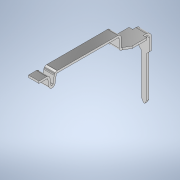
# Autodesk Inventor part: USB 3.0 A Recepticle Lower Pin
Saved by Autodesk Inventor 2020.1 (Build 241239000, 239)
## iProperties
Created: 2019-11-21
Part Number: USB 3.0 A Recepticle Lower Pin
Material: Nickel-Copper Alloy 400
Document SubType Name: Sheet Metal
Designer: S. Lee
Mass: 0.0317253 g
Surface Area: 0.43999 cm^2
Volume: 0.0035929 cm^3
Density: 8.83 g/cm^3
Appearance: Chrome - Polished
Flat Pattern Width: 0.17 cm
Flat Pattern Length: 1.89049 cm
Flat Pattern Area: 0.321383 cm^2
Sheet Metal Rule: Default_mm
Sheet Metal Width: 1.700 mm
Sheet Metal Length: 18.905 mm
Sheet Metal Area: 32.138 mm^2
Author: S. Lee
Autodesk Inventor part; units mm, degrees
ref_plane "YZ Plane" through (0, 0, 0) normal (1, 0, 0) x (0, 1, 0)
ref_plane "XZ Plane" through (0, 0, 0) normal (0, 1, 0) x (-1, 0, 0)
sketch "Sketch1" plane through (0, 0, 0) normal (1, 0, 0) x (0, 1, 0)
  line L0 (1.1156, 6.8012) -> (0.4531, 6.6963)
  line L1 (0.4531, 6.1037) -> (1.1156, 5.9988)
  line L2 (1.2, 5.9) -> (1.2, 0.1)
  line L3 (1.1, 0) -> (0.3, 0)
  line L4 (0, -0.3) -> (0, -2.6)
  line L5 (-0.3, -2.9) -> (-5.95, -2.9)
  line L6 (-5.95, -2.9) -> (-5.95, -3.1)
  line L7 (-5.95, -3.1) -> (-0.3, -3.1)
  line L8 (0.2, -2.6) -> (0.2, -0.3)
  line L9 (0.3, -0.2) -> (1.1, -0.2)
  line L10 (1.4, 0.1) -> (1.4, 5.9)
  line L11 (1.1469, 6.1963) -> (0.4844, 6.3012)
  line L12 (0.4844, 6.4988) -> (1.1469, 6.6037)
  line L13 (1.4, 6.9) -> (1.4, 7.65)
  line L14 (1.4, 7.65) -> (1.2, 7.65)
  line L15 (1.2, 7.65) -> (1.2, 6.9)
  line L16 (0, -5.3743) -> (0, 9.8207) projected
  line L17 (-7.4324, 0) -> (2.9446, 0) projected
  arc A0 (0.3, -0.2) -> (0.2, -0.3) centre (0.3, -0.3) ccw
  arc A1 (-0.3, -2.9) -> (0, -2.6) centre (-0.3, -2.6) ccw
  arc A2 (1.1, 0) -> (1.2, 0.1) centre (1.1, 0.1) ccw
  arc A3 (1.2, 5.9) -> (1.1156, 5.9988) centre (1.1, 5.9) ccw
  arc A4 (0.4844, 6.4988) -> (0.4844, 6.3012) centre (0.5, 6.4) ccw
  arc A5 (1.1156, 6.8012) -> (1.2, 6.9) centre (1.1, 6.9) ccw
  arc A6 (0.4531, 6.6963) -> (0.4531, 6.1037) centre (0.5, 6.4) ccw
  arc A7 (1.4, 5.9) -> (1.1469, 6.1963) centre (1.1, 5.9) ccw
  arc A8 (1.1469, 6.6037) -> (1.4, 6.9) centre (1.1, 6.9) ccw
  arc A9 (1.1, -0.2) -> (1.4, 0.1) centre (1.1, 0.1) ccw
  arc A10 (0.3, 0) -> (0, -0.3) centre (0.3, -0.3) ccw
  arc A11 (-0.3, -3.1) -> (0.2, -2.6) centre (-0.3, -2.6) ccw
  point P0 (1.2, 6.8146)
  point P1 (0, -2.9)
  point P2 (1.4, 6.1562)
  point P3 (-0.1393, 6.4)
  point P4 (1.4, 6.6438)
  dimension "d0" = 0.2
  dimension "d1" = 0.2
  dimension "d3" = 0.2
  dimension "d8" = 0.2
  dimension "d9" = 0.2
  dimension "d10" = 0.2
  dimension "d12" = 5.95
  dimension "d16" = 1.2
  dimension "d20" = 0.2438
  dimension "d21" = 0.2438
  dimension "d23" = 0.1
  dimension "d25" = 1
  dimension "d26" = 9.8
  dimension "d27" = 0.75
  dimension "d28" = 2.6
  dimension "d31" = 9.3
  dimension "d70" = 0.3
  constraints: 32 end point, 24 point on circle, 18 tangent, 12 centre point, 10 point on line, 7 parallel, 6 concentric, 5 perpendicular, 4 collinear, 4 equal radius
  measures "d0" distance between parallel lines of L4 L8
  measures "d1" distance between parallel lines of L7 L5
  measures "d3" distance between parallel lines of L9 L3
  measures "d8" distance between parallel lines of L1 L11
  measures "d9" distance between parallel lines of L10 L2
  measures "d10" distance between parallel lines of L0 L12
  measures "d12" distance between parallel lines of L6 L4
  measures "d16" distance between parallel lines of L4 L2
  measures "d20" vertical distance of point (-0.139, 6.4) point (1.4, 6.644)
  measures "d21" vertical distance of point (1.4, 6.156) point (-0.139, 6.4)
  measures "d23" radius of A0
  measures "d26" distance from line of L5 L15.end
  measures "d27" distance of L14.end L15.end
  measures "d28" vertical distance of L5.start L8.end
  measures "d31" distance from line of L5 A6.centre
  measures "d70" radius of A1
extrude "Extrusion1" add sketch "Sketch1" along normal blind 1.7 contours A5 L15 L14 L13 A8 L12 A4 L11 A7 L10 A9 L17 A2 L2 A3 L1 A6 L0 | L17 A9 L9 A0 L8 A11 L16 L4 A10 L3 | L16 A11 L7 L6 L5 A1
ref_plane "Work Plane1" through (0, 0.2, -0.3) normal (0, 0, 1) x (1, 0, 0)
sketch "Sketch2" plane through (0, 0.3, -0.3) normal (0, 0, -1) x (-1, 0, 0)
  line L0 (0, 1.1) -> (-1.7, 1.1) projected
  line L1 (0, -0.3) -> (-1.7, -0.3) projected
  line L2 (-1.35, 1.1) -> (-0.35, 1.1)
  line L3 (-0.35, 1.1) -> (-0.35, -0.3)
  line L4 (-0.35, -0.3) -> (-1.35, -0.3)
  line L5 (-1.35, -0.3) -> (-1.35, 1.1)
  line L6 (-1.7, 0) -> (-1.7, 0.8) projected
  line L7 (0, 0) -> (0, 0.8) projected
  line L8 (-1.7, 0) -> (-1.7, -0.3) projected
  line L9 (-1.35, 1.1) -> (-1.7, 1.1)
  line L10 (-1.7, 1.1) -> (-1.7, -0.3)
  line L11 (-1.7, -0.3) -> (-1.35, -0.3)
  line L12 (-1.35, -0.3) -> (-1.35, 1.1)
  line L13 (0, 0) -> (0, -0.3) projected
  line L14 (-0.35, 1.1) -> (0, 1.1)
  line L15 (0, 1.1) -> (0, -0.3)
  line L16 (0, -0.3) -> (-0.35, -0.3)
  line L17 (-0.35, -0.3) -> (-0.35, 1.1)
  dimension "d32" = 1
  dimension "d33" = 0.35
  dimension "d34" = 0.35
  constraints: 24 end point, 6 parallel, 3 horizontal, 3 perpendicular, 2 point on line
  measures "d32" distance of L3.end L4.end
  measures "d33" distance between parallel lines of L6 L5
  measures "d34" distance between parallel lines of L7 L3
extrude "Extrusion2" cut sketch "Sketch2" against normal up to surface (7.95 mm away) contours L15 L7 L13 L1 L3 L0 | L5 L1 L8 L6 L10 L0
sketch "Sketch3" plane through (0, 0.2, -2.6) normal (0, 1, 0) x (1, 0, 0)
  line L0 (0.35, -2.3) -> (1.35, -2.3) projected
  line L1 (1.35, -2.3) -> (1.7, -1.6938)
  line L2 (1.7, 0) -> (1.7, -2.3) projected
  line L3 (1.35, -2.3) -> (2.05, -2.3) construction
  line L4 (1.7, -1.6938) -> (1.7, -2.3)
  line L5 (1.35, -2.3) -> (1.7, -2.3) projected
  line L6 (1.7, -2.3) -> (1.35, -2.3)
  line L7 (1.35, -2.3) -> (0.35, -2.3)
  line L8 (0, -2.3) -> (0, 0) projected
  line L9 (0.35, -2.3) -> (0, -2.3)
  line L10 (0, -2.3) -> (0, -1.6938)
  line L11 (0, -1.6938) -> (0.35, -2.3)
  line L12 (0.35, -0.3) -> (0.35, 0.3)
  line L13 (1.35, -0.3) -> (1.7, -0.3)
  line L14 (1.7, -0.3) -> (1.7, 0.5)
  line L15 (1.7, 0.5) -> (1.35, 0.5)
  line L16 (1.35, 0.5) -> (1.35, -0.3)
  line L17 (0.35, -0.3) -> (0, -0.3)
  line L18 (0, -0.3) -> (0, 0.5)
  line L19 (0, 0.5) -> (0.35, 0.5)
  line L20 (0.35, 0.5) -> (0.35, -0.3)
  line L21 (0, 0) -> (1.7, 0) projected
  point P0 (0, -2.6)
  point P1 (0, -1.6938)
  point P2 (0.35, 0.3)
  point P3 (0.35, 0.3)
  dimension "d38" = 60
  dimension "d39" = 60
  dimension "d59" = 2
  dimension "d60" = 2
  dimension "d62" = 1
  dimension "d63" = 0.35
  dimension "d64" = 0.35
  constraints: 34 end point, 4 parallel, 4 perpendicular, 3 horizontal, 2 collinear, 1 equal length, 1 point on line, 1 vertical
  measures "d38" angle of L3 L1
  measures "d39" angle of L11 L9
  measures "d59" distance between parallel lines of L17 L0
  measures "d60" distance between parallel lines of L13 L0
  measures "d62" distance between parallel lines of L16 L20
  measures "d63" distance between parallel lines of L12 L18
  measures "d64" distance between parallel lines of L16 L14
extrude "Extrusion3" cut sketch "Sketch3" against normal up to surface (6.15 mm away) contours L9 L8 L11 | L1 L2 L5 | L8 L21 L12 L17 | L13 L16 L21 L2 | L18 L19 L20 L12 L21 | L21 L16 L15 L14
sketch "Sketch5" plane through (1.35, -0.3, -3.1) normal (0, 0, -1) x (-1, 0, 0)
  line L0 (0, -1.15) -> (0.25, -1.4)
  line L1 (0.25, -1.4) -> (0.25, -5.317)
  line L2 (0.25, -5.317) -> (0.4134, -5.6)
  line L3 (0.5866, -5.6) -> (0.75, -5.317)
  line L4 (0.75, -5.317) -> (0.75, -1.4)
  line L5 (0.75, -1.4) -> (1, -1.15)
  line L6 (0.25, -5.317) -> (0.75, -5.317) construction
  line L7 (0, -1.15) -> (1, -1.15) construction
  arc A0 (0.4134, -5.6) -> (0.5866, -5.6) centre (0.5, -5.55) ccw
  line L8 (0, 0.3) -> (-0.35, 0.3) projected
  line L9 (1.35, 0.3) -> (1, 0.3) projected
  line L10 (0, 0) -> (0, -5.65) projected
  line L11 (1, -5.65) -> (1, 0) projected
  line L12 (1, -5.65) -> (0, -5.65) projected
  point P0 (0.5, -5.65)
  point P1 (1.35, -5.85)
  point P2 (-0.35, -5.85)
  point P3 (0, 0.6)
  point P4 (1, 0.6)
  point P5 (0.5, -5.35)
  dimension "d45" = 60
  dimension "d46" = 0.5
  dimension "d48" = 135
  dimension "d49" = 135
  dimension "d53" = 0.1
  dimension "d65" = 1.7
  dimension "d66" = 1.7
  dimension "d67" = 0.25
  dimension "d68" = 0.5
  dimension "d69" = 0.25
  constraints: 16 end point, 2 parallel, 2 point on circle, 2 tangent, 1 centre point, 1 point on line, 4 other
  measures "d45" angle of L3 L2
  measures "d46" distance between parallel lines of L4 L1
  measures "d48" angle of L0 L1
  measures "d49" angle of L4 L5
  measures "d53" radius of A0
  measures "d67" distance between parallel lines of L10 L1
  measures "d68" distance from line of L11 A0.centre
  measures "d69" distance from line of L7 L0.end
extrude "Extrusion4" cut sketch "Sketch5" against normal up to surface (0.2 mm away)
equation "\"d20\" = d21"
equation "\"d33\" = d34"
equation "\"d63\" = d64"
equation "\"BendRadius\" = Thickness"
equation "\"BendReliefWidth\" = Thickness"
equation "\"BendReliefDepth\" = 0.5 * Thickness"
equation "\"CornerReliefSize\" = 4 * Thickness"
equation "\"MinimumRemnant\" = 2 * Thickness"
equation "\"TransitionRadius\" = BendRadius"
equation "\"JacobiRadiusSize\" = BendRadius"
equation "\"GapSize\" = Thickness"
equation "\"Thickness\" = 0.2"
body "Solid1"
